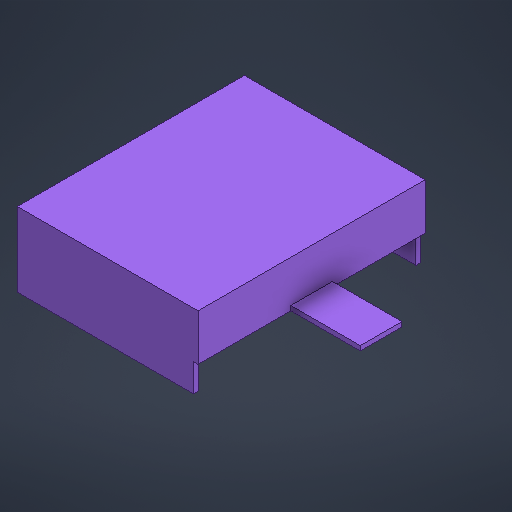
# Autodesk Inventor part: Víko senzor
Saved by Autodesk Inventor 2026.2 (Build 302298000, 298)
## iProperties
Created: 2026-03-13
Part Number: Víko senzor
Material: Všeobecné
Document SubType Name: Modeling
Designer: cerna
Density: 1 g/cm^3
Appearance: Fialová
Author: cerna
Autodesk Inventor part; units mm, degrees
ref_plane "YZ Plane" through (0, 0, 0) normal (1, 0, 0) x (0, 1, 0)
ref_plane "XZ Plane" through (0, 0, 0) normal (0, 1, 0) x (-1, 0, 0)
ref_plane "XY Plane" through (0, 0, 0) normal (0, 0, 1) x (1, 0, 0)
sketch "Náčrt1" plane through (0, 0, 0) normal (0, 1, 0) x (-1, 0, 0)
  line L0 (7.7382, 6.9283) -> (7.7382, -42.0717)
  line L1 (7.7382, -42.0717) -> (-31.2618, -42.0717)
  line L2 (-31.2618, -42.0717) -> (-31.2618, 6.9283)
  line L3 (-31.2618, 6.9283) -> (7.7382, 6.9283)
  line L4 (6.7382, -41.0717) -> (6.7382, 5.9283)
  line L5 (6.7382, 5.9283) -> (-30.2618, 5.9283)
  line L6 (-30.2618, 5.9283) -> (-30.2618, -41.0717)
  line L7 (-30.2618, -41.0717) -> (6.7382, -41.0717)
  point P0 (0, 0)
  dimension "d0" = 49
  dimension "d1" = 39
  dimension "d2" = 1
  constraints: 16 end point, 4 perpendicular, 2 parallel, 1 vertical, 3 other
  measures "d0" distance of L0.start L0.end
  measures "d1" distance of L0.end L1.end
  measures "d2" distance between parallel lines of L0 L4
extrude "Vysunutí1" add sketch "Náčrt1" along normal blind 15
sketch "Náčrt2" plane through (0, 15, 0) normal (0, 1, 0) x (1, 0, 0)
  line L0 (31.2618, -6.9283) -> (31.2618, 42.0717) projected
  line L1 (31.2618, 42.0717) -> (-7.7382, 42.0717) projected
  line L2 (-7.7382, 42.0717) -> (-7.7382, -6.9283) projected
  line L3 (-7.7382, -6.9283) -> (31.2618, -6.9283) projected
  line L4 (-6.7382, 41.0717) -> (30.2618, 41.0717) projected
  line L5 (30.2618, 41.0717) -> (30.2618, -5.9283) projected
  line L6 (30.2618, -5.9283) -> (-6.7382, -5.9283) projected
  line L7 (-6.7382, -5.9283) -> (-6.7382, 41.0717) projected
  line L8 (-7.7382, -6.9283) -> (31.2618, -6.9283)
  line L9 (31.2618, -6.9283) -> (31.2618, 42.0717)
  line L10 (31.2618, 42.0717) -> (-7.7382, 42.0717)
  line L11 (-7.7382, 42.0717) -> (-7.7382, -6.9283)
  point P0 (0, 0)
  constraints: 8 end point, 2 parallel, 1 horizontal, 1 perpendicular
extrude "Vysunutí2" add sketch "Náčrt2" along normal blind 1 contours L3 L2 L1 L0 | L4 L5 L6 L7
sketch "Náčrt3" plane through (31.2618, 0, 6.9283) normal (1, 0, 0) x (0, 0, -1)
  line L0 (0, 0) -> (49, 0) projected
  line L1 (49, 0) -> (49, 16) projected
  line L2 (0, 16) -> (49, 16) projected
  line L3 (0, 0) -> (0, 16) projected
  line L4 (0, 0) -> (49, 0)
  line L5 (49, 0) -> (49, 6)
  line L6 (49, 6) -> (0, 6)
  line L7 (0, 6) -> (0, 0)
  point P0 (6.9283, 0)
  point P1 (0, 6)
  dimension "d7" = 6
  constraints: 8 end point, 2 parallel, 1 horizontal, 1 perpendicular, 1 point on line
  measures "d7" distance between parallel lines of L6 L0
extrude "Vysunutí3" cut sketch "Náčrt3" against normal blind 1 contours L3 L6 L1 L0
sketch "Náčrt4" plane through (31.2618, 16, 6.9283) normal (1, 0, 0) x (0, 0, -1)
  line L0 (0, -10) -> (49, -10) projected
  line L1 (49, -10) -> (49, 0) projected
  line L2 (0, 0) -> (49, 0) projected
  line L3 (0, -10) -> (0, 0) projected
  line L4 (20, -10) -> (29, -10)
  line L5 (29, -10) -> (29, -9)
  line L6 (29, -9) -> (20, -9)
  line L7 (20, -9) -> (20, -10)
  point P0 (6.9283, -16)
  dimension "d10" = 20
  dimension "d11" = 1
  dimension "d12" = 20
  constraints: 8 end point, 2 parallel, 1 horizontal, 1 perpendicular, 1 point on line
  measures "d10" distance between parallel lines of L7 L3
  measures "d11" distance between parallel lines of L0 L6
  measures "d12" distance between parallel lines of L1 L5
extrude "Vysunutí4" add sketch "Náčrt4" along normal blind 15 contours L7 L6 L5 L0
